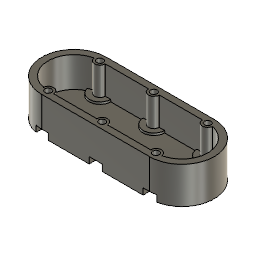
Robosoc_motor_case_top (Autodesk Fusion 360 design; units mm, degrees)
part number: 2025-11-26-14-21-49-432
Autodesk Fusion 360 part; units mm, degrees
note: some values were not read from the file. Set by a fixed rule: which sketch regions a step uses.
sketch "Sketch1" plane through (0, 0, 0) normal (0, 0, 1) x (1, 0, 0)
  line L0 (15, 0) -> (65.0001, 0)
  line L1 (65.0001, 30) -> (15, 30)
  arc A0 (65.0001, 0) -> (65.0001, 30) centre (65, 15) ccw
  arc A1 (15, 30) -> (15, 0) centre (15, 15) ccw
  line L2 (0, 0) -> (0, 40.5539) construction
  line L3 (0, 0) -> (80, 0) construction
  dimension "d9" = 15
  dimension "d10" = 50
  constraint horizontal L0
  constraint horizontal L1
  constraint tangent L1 A1
  constraint tangent L0 A1
  constraint equal A0 A1
  constraint coincident L2.start L3.start
  constraint vertical L2
  constraint tangent A1 L2
  constraint perpendicular L2 L3
  constraint collinear L0 L3
  measures "d9" radius of A0
  measures "d10" distance of A0.centre A1.centre
extrude "Extrude1" add sketch "Sketch1" along normal blind 3
sketch "Sketch2" plane through (0, 0, 3) normal (0, 0, 1) x (-1, 0, 0)
  arc A0 (-15, -30) -> (-15, 0) centre (-15, -15) ccw
  line L0 (-15, 0) -> (-65.0001, 0)
  arc A1 (-65.0001, 0) -> (-65.0001, -30) centre (-65, -15) ccw
  line L1 (-65.0001, -30) -> (-15, -30)
  arc A2 (-65.0001, -3) -> (-65, -27) centre (-65, -15) ccw
  line L2 (-65, -27) -> (-15, -27)
  arc A3 (-15, -27) -> (-15, -3) centre (-15, -15) ccw
  line L3 (-15, -3) -> (-65.0001, -3)
  line L4 (-65, -15) -> (-65.0001, 0) construction
  line L5 (-65.0001, 0) -> (-15.0001, 0.0002) construction
  line L6 (-15.0001, 0.0002) -> (-15, -15) construction
  line L7 (-15, -15) -> (-65, -15) construction
  arc A4 (-69.8903, -4.0417) -> (-60.0001, -3) centre (-65.0001, -3) ccw
  arc A5 (-45, -3) -> (-35, -3) centre (-40, -3.0001) ccw
  arc A6 (-20, -3) -> (-10.1097, -4.0417) centre (-15, -3) ccw
  arc A7 (-18.9998, 0.0002) -> (-19, 0) centre (-15, -3) ccw
  arc A8 (-20, -3) -> (-10.1097, -4.0417) centre (-15, -3) ccw
  arc A9 (-45, -3) -> (-35, -3) centre (-40, -3.0001) ccw
  arc A10 (-69.8903, -4.0417) -> (-60.0001, -3) centre (-65.0001, -3) ccw
  line L8 (-15.0001, -14.9998) -> (-15, -30) construction
  line L9 (-15, -30) -> (-15.9207, -30) construction
  line L10 (-15, -30) -> (-65, -30) construction
  arc A11 (-35, -27) -> (-45, -27) centre (-40, -27) ccw
  arc A12 (-10.1097, -25.9583) -> (-20, -27) centre (-15, -27) ccw
  arc A13 (-60, -27) -> (-69.8903, -25.9583) centre (-65, -27) ccw
  circle A14 centre (-15, -27) radius 1.5
  circle A15 centre (-40, -27) radius 1.5
  circle A16 centre (-65, -27) radius 1.5
  circle A17 centre (-15, -3) radius 1.5
  circle A18 centre (-40, -3) radius 1.5
  circle A19 centre (-65, -3) radius 1.5
  circle A20 centre (-40, -3) radius 2.5
  circle A21 centre (-65, -3) radius 2.5
  circle A22 centre (-65, -27) radius 2.5
  circle A23 centre (-40, -27) radius 2.5
  circle A24 centre (-15, -27) radius 2.5
  circle A25 centre (-15, -3) radius 2.5
  dimension "d13" = -3
  dimension "d44" = 10
  dimension "d47" = 10
  dimension "d48" = 10
  dimension "d51" = 10
  dimension "d52" = 10
  dimension "d53" = 10
  dimension "d55" = 10
  dimension "d56" = 10
  dimension "d57" = 10
  dimension "d60" = 3
  dimension "d61" = 3
  dimension "d62" = 3
  dimension "d63" = 3
  dimension "d64" = 3
  dimension "d65" = 3
  dimension "d66" = 1
  dimension "d67" = 1
  dimension "d68" = 1
  dimension "d69" = 1
  dimension "d70" = 1
  dimension "d71" = 1
  constraint coincident A1.centre A2.centre
  constraint coincident L0.end A1.start
  constraint perpendicular L4 L5
  constraint coincident A0.centre A3.centre
  constraint coincident A2.start L3.end
  constraint coincident L3 A4.end
  constraint coincident A2 A4.start
  constraint coincident A3.end L3.start
  constraint coincident L3 A5.end
  constraint coincident L3 A5.start
  constraint coincident L0 A7.end
  constraint coincident L3 A6.start
  constraint coincident L5 A7.start
  constraint concentric A6 A7
  constraint coincident A3 A6.end
  constraint coincident A0.start L1.end
  constraint coincident L1 L9.end
  constraint parallel L1 L10
  constraint coincident L2.end A3.start
  constraint coincident L2 A11.end
  constraint coincident L2 A11.start
  constraint coincident A3 A12.start
  constraint coincident L2 A12.end
  constraint coincident L2 A13.start
  constraint coincident A2 A13.end
  constraint concentric A12 A14
  measures "d44" diameter of A4
  measures "d47" diameter of A6
  measures "d48" diameter of A5
  measures "d51" diameter of A10
  measures "d52" diameter of A8
  measures "d53" diameter of A9
  measures "d55" diameter of A12
  measures "d56" diameter of A11
  measures "d57" diameter of A13
  measures "d60" diameter of A14
  measures "d61" diameter of A15
  measures "d62" diameter of A16
  measures "d63" diameter of A17
  measures "d64" diameter of A18
  measures "d65" diameter of A19
extrude "Extrude2" add sketch "Sketch2" along normal blind 14 contours A0 L0 A1 L1 A2 L2 A3 L3 A7 A20 A21 A22 A23 A24 | A0 L0 A3 L3 A7 A25 | A3 L3 A17 A25 | L2 A3 A14 A24 | A3 L3 A17 | L3 A18 A20 | L2 A3 A14 | L3 A18 | L2 A15 A23 | A2 L3 A19 A21 | L2 A15 | A2 L3 A19 | A2 L2 A16 A22 | A2 L2 A16 picked at (-13.0721, -2.848) picked at (-13.0721, -27.152) picked at (-14.6506, -2.538) picked at (-42.1518, -2.8013) picked at (-14.6506, -27.462) picked at (-40.339, -2.2448) picked at (-42.1518, -27.1987) picked at (-66.9146, -2.7753) picked at (-39.7775, -27.9749) picked at (-65.3253, -2.5293) picked at (-66.9146, -27.2247) picked at (-65.3252, -27.4707)
sketch "Sketch3" plane through (0, 0, 0) normal (0, 0, -1) x (1, 0, 0)
  arc A0 (15, 0) -> (15, -30) centre (15, -15) ccw
  line L0 (15, -30) -> (65.0001, -30)
  arc A1 (65.0001, -30) -> (65.0001, 0) centre (65, -15) ccw
  line L1 (65.0001, 0) -> (15, 0)
  line L2 (65, -15) -> (65.0001, 0) construction
  line L3 (65, -15) -> (15, -15) construction
  line L4 (15, -15) -> (15, 0) construction
  line L5 (15, 0) -> (65.0001, 0) construction
  line L6 (15, 0) -> (15, -3) construction
  line L7 (18, -3) -> (18, 0) construction
  line L8 (18, 0) -> (12, 0) construction
  line L9 (12, 0) -> (12, -3) construction
  line L10 (12, -3) -> (12, 0) construction
  line L11 (15, 0) -> (18, 0) construction
  line L12 (18, 0) -> (18, -3) construction
  line L13 (12, -3) -> (12, 0)
  line L14 (12, 0) -> (18, 0)
  line L15 (18, 0) -> (18, -3)
  arc A2 (12, -3) -> (18, -3) centre (15, -3) ccw
  line L16 (40, -3) -> (43, -3) construction
  line L17 (43, 0) -> (37, 0) construction
  line L18 (37, 0) -> (43, 0)
  line L19 (43, 0) -> (43, -3)
  line L20 (37, -3) -> (37, 0)
  arc A3 (37, -2.998) -> (43, -3) centre (40, -3) ccw
  line L21 (65, -3) -> (68, -3) construction
  arc A4 (65.0066, 0) -> (64.9934, 0) centre (65, -3) ccw
  arc A5 (68, -27) -> (62, -27) centre (65, -27) ccw
  line L22 (62, -30) -> (62, -27)
  line L23 (68, -27) -> (68, -30)
  arc A6 (43, -27.002) -> (37, -27) centre (40, -27) ccw
  line L24 (43, -27) -> (43, -30)
  line L25 (37, -30) -> (37, -27)
  line L26 (18, -27) -> (18, -30)
  arc A7 (18, -27.0025) -> (12, -27) centre (15, -27) ccw
  line L27 (12, -30) -> (12, -27)
  line L28 (68, 0) -> (68, -3)
  arc A8 (62, -2.998) -> (68, -3) centre (65, -3) ccw
  line L29 (62, -3) -> (62, 0)
  line L30 (62, 0) -> (68, 0)
  dimension "d16" = 6
  dimension "d17" = 6
  dimension "d23" = 6
  dimension "d25" = 6
  dimension "d27" = 6
  dimension "d28" = 6
  dimension "d29" = 6
  dimension "d40" = 6
  constraint coincident A1.centre L2.start
  constraint coincident A1.end L1.start
  constraint coincident A0.centre L3.end
  constraint coincident A0.start L1.end
  constraint coincident L4 L6.end
  constraint tangent L5 A2
  constraint coincident L5 L7.end
  constraint perpendicular L5 L7
  constraint perpendicular L7 L8
  constraint coincident L9.end A2
  constraint tangent L9 A2
  constraint vertical L10
  constraint horizontal L11
  constraint vertical L12
  constraint vertical L13
  constraint horizontal L14
  constraint vertical L15
  constraint coincident L9 L10.start
  constraint coincident L16.start A3.centre
  constraint horizontal L16
  constraint coincident L5 L17.start
  constraint parallel L5 L17
  constraint horizontal L18
  constraint vertical L19
  constraint vertical L20
  constraint coincident L20 A3.start
  constraint perpendicular L2 L21
  constraint coincident L1 A4.end
  constraint coincident A1 A4.start
  constraint coincident A6.start L24
  constraint coincident L27.end A7
  constraint coincident A7.start L26
  constraint coincident A7.end L27
  constraint perpendicular L0 L22
  constraint perpendicular L0 L24
  constraint perpendicular L0 L25
  constraint perpendicular L0 L26
  constraint coincident L26.start A7
  constraint vertical L28
  constraint vertical L29
  constraint coincident A8.start L29
  constraint perpendicular L28 L30
  measures "d16" diameter of A2
  measures "d17" diameter of A3
  measures "d23" distance of L7.start L9.end
  measures "d25" distance of L17.start L17.end
  measures "d27" diameter of A5
  measures "d28" diameter of A6
  measures "d29" diameter of A7
  measures "d40" diameter of A8
extrude "Extrude3" cut sketch "Sketch3" against normal blind 3 contours A0 L1 L13 L14 L15 A2
extrude "Extrude4" cut sketch "Sketch3" against normal blind 3 contours L1 L18 L19 L20 A3
extrude "Extrude5" cut sketch "Sketch3" against normal blind 3 contours L0 A6 L24 L25
extrude "Extrude6" cut sketch "Sketch3" against normal blind 3 contours A0 L0 L26 A7 L27
extrude "Extrude7" cut sketch "Sketch3" against normal blind 3 contours L0 A1 A5 L22 L23
extrude "Extrude8" cut sketch "Sketch3" against normal blind 3 contours A1 L1 A4 L28 A8 L29 L30
extrude "Extrude9" add sketch "Sketch2" along normal blind 1 contours A2 L3 A4 A10 A21 | A2 L3 A19 A21 | A2 L3 A19 picked at (-66.8477, -3.5405) picked at (-65.3313, -3.4756)
extrude "Extrude10" add sketch "Sketch2" along normal blind 1 contours A3 L3 A6 A7 A8 A25 | A3 L3 A17 A25 | L3 A5 A9 A20 | A3 L3 A17 | L3 A18 A20 | L3 A18 picked at (-13.1523, -3.5405) picked at (-14.6688, -3.4756) picked at (-42.1574, -3.1242) picked at (-40.3832, -3.562)
extrude "Extrude11" add sketch "Sketch2" along normal blind 1 contours L2 A3 A12 A24 | L2 A3 A14 A24 | L2 A3 A14 | L2 A11 A23 | L2 A15 A23 | L2 A15 | A2 L2 A13 A22 | A2 L2 A16 A22 | A2 L2 A16 picked at (-13.1523, -26.4595) picked at (-14.6688, -26.5244) picked at (-42.1574, -26.8758) picked at (-39.6335, -26.6599) picked at (-66.8477, -26.4595) picked at (-65.3313, -26.5244)
extrude "Extrude12" add sketch "Sketch2" along normal blind 14 contours A3 L3 A17 A25 | A3 L3 A17 A25 | A3 L3 A17 | A3 L3 A17
extrude "Extrude13" cut sketch "Sketch2" along normal blind 15 contours A3 L3 A17 | A3 L3 A17
extrude "Extrude14" add sketch "Sketch2" along normal blind 14 contours A3 L3 A17 A25 | A3 L3 A17 A25 | L2 A3 A14 A24 | L2 A3 A14 A24 | A3 L3 A17 | A3 L3 A17 | L3 A18 A20 | L3 A18 A20 | L2 A3 A14 | L2 A3 A14 | L3 A18 | L3 A18 | L2 A15 A23 | L2 A15 A23 | A2 L3 A19 A21 | A2 L3 A19 A21 | L2 A15 | L2 A15 | A2 L3 A19 | A2 L3 A19
extrude "Extrude15" add sketch "Sketch2" along normal blind 14 contours A2 L2 A16 A22 | A2 L2 A16 A22 | A2 L2 A16 | A2 L2 A16
extrude "Extrude16" cut sketch "Sketch2" along normal blind 15 contours A3 L3 A17 | A3 L3 A17 | L2 A3 A14 | L2 A3 A14 | L3 A18 | L3 A18 | L2 A15 | L2 A15 | A2 L3 A19 | A2 L3 A19 | A2 L2 A16 | A2 L2 A16
